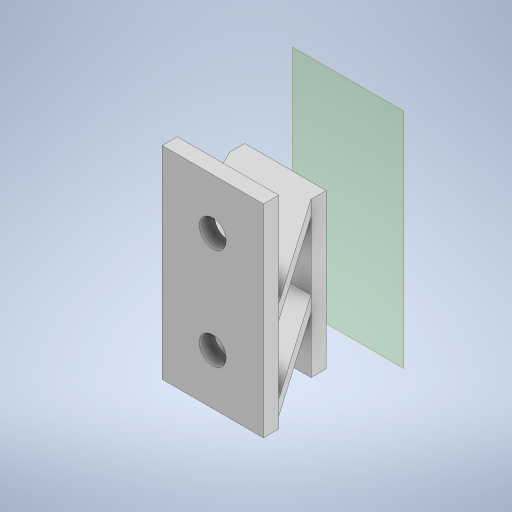
# Autodesk Inventor part: Soporte X
Saved by Autodesk Inventor 2024 (Build 280153000, 153)
## iProperties
Created: 2024-06-03
Part Number: Soporte X
Material: Generic
Document SubType Name: Modeling
Designer: juanp
Density: 1 g/cm^3
Appearance: Default
Author: juanp
Autodesk Inventor part; units mm, degrees
ref_plane "YZ Plane" through (0, 0, 0) normal (1, 0, 0) x (0, 1, 0)
ref_plane "XZ Plane" through (0, 0, 0) normal (0, 1, 0) x (-1, 0, 0)
ref_plane "XY Plane" through (0, 0, 0) normal (0, 0, 1) x (1, 0, 0)
sketch "Sketch1" plane through (0, 0, 0) normal (0, 0, 1) x (1, 0, 0)
  line L0 (10, -20) -> (-10, -20)
  line L1 (-10, -20) -> (-10, 20)
  line L2 (-10, 20) -> (10, 20)
  line L3 (10, 20) -> (10, -20)
  line L4 (10, -20) -> (-10, 20) construction
  line L5 (-10, -20) -> (10, 20) construction
  line L6 (0, -10) -> (0, 10) construction
  circle A0 centre (0, 10) radius 2.65
  circle A1 centre (0, -10) radius 2.65
  point P0 (0, 0)
  dimension "d0" = 40
  dimension "d1" = 20
  dimension "d2" = 20
  dimension "d3" = 5.3
  constraints: 14 end point, 3 midpoint, 2 centre point, 2 coincident, 2 parallel, 1 equal radius, 1 horizontal, 1 perpendicular, 1 vertical
  measures "d0" distance between parallel lines of L2 L0
  measures "d1" distance of L1.end L2.end
  measures "d2" distance of L6.start L6.end
  measures "d3" diameter of A0
extrude "Extrusion1" add sketch "Sketch1" along normal blind 3
ref_plane "Work Plane2" through (0, 0, -24) normal (0, 0, -1) x (-1, 0, 0)
sketch "Sketch2" plane through (0, 0, -24) normal (0, 0, -1) x (-1, 0, 0)
  circle A0 centre (18.05, -6.8) radius 1.65
  line L0 (18.05, -25.9) -> (18.05, -6.8) construction
  line L1 (4.6, -29) -> (20.7, -29)
  line L2 (4.6, 11.5) -> (4.6, -29)
  line L3 (20.7, 11.5) -> (4.6, 11.5)
  line L4 (20.7, -29) -> (20.7, 11.5)
  circle A1 centre (18.05, -25.9) radius 1.65
  line L5 (10, 20) -> (10, -20) projected
  line L6 (-10, 20) -> (10, 20) projected
  point P0 (0, 0)
  dimension "d8" = 40.5
  dimension "d9" = 16.1
  dimension "d10" = 19.1
  dimension "d11" = 3.3
  dimension "d12" = 3.3
  dimension "d13" = 2.65
  dimension "d14" = 3.1
  dimension "d15" = 8.05
  dimension "d19" = 26.8
  constraints: 10 end point, 2 centre point, 2 coincident, 2 parallel, 1 perpendicular, 1 vertical
  measures "d8" distance of L3.start L4.start
  measures "d9" distance of L3.start L2.start
  measures "d10" distance of L0.start L0.end
  measures "d11" diameter of A1
  measures "d12" diameter of A0
  measures "d13" distance between parallel lines of L0 L4
  measures "d14" distance from line of L0.start L1
  measures "d15" distance from line of L5 L0.end
  measures "d19" distance from line of L6 L0.end
extrude "Extrusion2" add sketch "Sketch2" against normal blind 3
sketch "Sketch4" plane through (0, 0, -21) normal (0, 0, 1) x (1, 0, 0)
  line L0 (-20.7, -14.85) -> (-4.6, -14.85)
  line L1 (-4.6, -14.85) -> (-4.6, -17.85)
  line L2 (-4.6, -17.85) -> (-20.7, -17.85)
  line L3 (-20.7, -17.85) -> (-20.7, -14.85)
  line L4 (-4.6, 1.5) -> (-20.7, 1.5)
  line L5 (-20.7, 1.5) -> (-20.7, -1.5)
  line L6 (-20.7, -1.5) -> (-4.6, -1.5)
  line L7 (-4.6, -1.5) -> (-4.6, 1.5)
  line L8 (-20.7, -16.35) -> (-4.6, -16.35) construction
  circle A0 centre (-18.05, -6.8) radius 1.65 projected
  circle A1 centre (-18.05, -25.9) radius 1.65 projected
  line L9 (-18.05, -6.8) -> (-18.05, -25.9) construction
  line L10 (-4.6, -29) -> (-4.6, 11.5) projected
  line L11 (-20.7, 11.5) -> (-20.7, -29) projected
  line L12 (-20.7, 0) -> (-4.6, 0) construction
  line L13 (-10, 20) -> (-10, -20) projected
  point P0 (0, 0)
  point P1 (-18.05, -16.35)
  point P2 (-10, 0)
  dimension "d20" = 3
  constraints: 22 end point, 6 midpoint, 6 point on line, 4 parallel, 3 horizontal, 2 perpendicular, 1 collinear, 1 vertical
  measures "d20" distance of L4.end L5.end
sketch "Sketch5" plane through (0, 0, 0) normal (0, 0, -1) x (-1, 0, 0)
  line L0 (4.6, 1.5) -> (20.7, 1.5) projected
  line L1 (20.7, -1.5) -> (4.6, -1.5) projected
  line L2 (4.6, -17.85) -> (20.7, -17.85) projected
  line L3 (20.7, -14.85) -> (4.6, -14.85) projected
  line L4 (-10, 1.5) -> (10, 1.5)
  line L5 (10, 1.5) -> (10, -1.5)
  line L6 (10, -1.5) -> (-10, -1.5)
  line L7 (-10, -1.5) -> (-10, 1.5)
  line L8 (-10, -14.85) -> (10, -14.85)
  line L9 (10, -14.85) -> (10, -17.85)
  line L10 (10, -17.85) -> (-10, -17.85)
  line L11 (-10, -17.85) -> (-10, -14.85)
  line L12 (-10, -20) -> (-10, 20) projected
  line L13 (10, 20) -> (10, -20) projected
  point P0 (0, 0)
  constraints: 16 end point, 4 collinear, 4 parallel, 4 point on line, 2 horizontal, 2 perpendicular
loft "Loft1" add profiles "Sketch4", "Sketch5" contours L5 L4 L13 L6 | L13 L4 L7 L6 / L0 L5 L1 L6 L7 L4
loft "Loft2" add profiles "Sketch4", "Sketch5" contours L0 L13 L2 L3 | L0 L1 L2 L13 / L9 L2 L10 L11 L8 L3
sketch "Sketch6" plane through (0, 0, -21) normal (0, 0, 1) x (1, 0, 0)
  line L0 (-20.7, 1.5) -> (-4.6, 1.5) projected
  line L1 (-4.6, 1.5) -> (-4.6, 11.5) projected
  line L2 (-4.6, 11.5) -> (-20.7, 11.5) projected
  line L3 (-20.7, 11.5) -> (-20.7, 1.5) projected
  point P0 (0, 0)
extrude "Extrusion3" cut sketch "Sketch6" against normal through all
body "Solid1"
